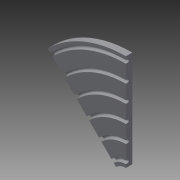
# Autodesk Inventor part: Curved Track Builder
Saved by Autodesk Inventor 2015 SP1 (Build 190203100, 203)
## iProperties
Created: 2015-05-26
Part Number: Curved Track Builder
Material: Generic
Document SubType Name: Modeling
Designer: Andrew
Density: 1 g/cm^3
Appearance: Default
Author: Andrew
Autodesk Inventor part; units mm, degrees
ref_plane "YZ Plane" through (0, 0, 0) normal (1, 0, 0) x (0, 1, 0)
ref_plane "XZ Plane" through (0, 0, 0) normal (0, 1, 0) x (-1, 0, 0)
ref_plane "XY Plane" through (0, 0, 0) normal (0, 0, 1) x (1, 0, 0)
sketch "Sketch1" plane through (0, 0, 0) normal (0, 1, 0) x (-1, 0, 0)
  arc A0 (77.046154, 77.046154) -> (0, 108.959716) centre (0, 0) ccw
  arc A1 (64.375202, 64.375202) -> (0, 91.040284) centre (0, 0) ccw
  line L0 (0, 113.959716) -> (0, 0)
  arc A2 (51.70425, 51.70425) -> (0, 73.120851) centre (0, 0) ccw
  arc A3 (39.033297, 39.033297) -> (0, 55.201418) centre (0, 0) ccw
  arc A4 (26.362345, 26.362345) -> (0, 37.281986) centre (0, 0) ccw
  arc A5 (70.710678, 70.710678) -> (0, 100) centre (0, 0) ccw construction
  arc A6 (13.691392, 13.691392) -> (0, 19.362553) centre (0, 0) ccw
  line L1 (0, 0) -> (80.581688, 80.581688)
  arc A7 (80.581688, 80.581688) -> (0, 113.959716) centre (0, 0) ccw
  arc A8 (10.155859, 10.155859) -> (0, 14.362553) centre (0, 0) ccw
  dimension "d8" = 45
  dimension "d0" = 17.91943
  dimension "d2" = 8.95972
  dimension "d3" = 200
  dimension "d4" = 17.91943
  dimension "d5" = 17.91943
  dimension "d6" = 17.91943
  dimension "d9" = 17.91943
  dimension "d10" = 5
  dimension "d11" = 5
  constraints: 18 point on circle, 9 centre point, 9 coincident, 21 other
  measures "d0" radial gap between concentric circles of A0 A1
  measures "d2" radial gap between concentric circles of A5 A1
  measures "d3" diameter of A5
  measures "d4" radial gap between concentric circles of A2 A1
  measures "d5" radial gap between concentric circles of A3 A2
  measures "d6" radial gap between concentric circles of A3 A4
  measures "d9" radial gap between concentric circles of A6 A4
  measures "d10" radial gap between concentric circles of A8 A6
  measures "d11" radial gap between concentric circles of A7 A0
extrude "Extrusion1" add sketch "Sketch1" along normal blind 5 contours L1 A1 L0 A0 | A0 L0 A7 L1 | L1 A2 L0 A1 | L1 A3 L0 A2 | L1 A4 L0 A3 | L1 A6 L0 A4 | L1 A8 L0 A6
sketch "Sketch2" plane through (-80.581688, 0, 80.581688) normal (-0.7071068, 0, -0.7071068) x (-0.7071068, 0, 0.7071068)
  line L0 (-5, 0) -> (-36.913562, 0)
  line L1 (-22.919433, 0) -> (-49.584514, 0)
  line L2 (-40.838865, 0) -> (-62.255467, 0)
  line L3 (-58.758298, 0) -> (-74.926419, 0)
  line L4 (-76.677731, 0) -> (-87.597372, 0)
  line L5 (-94.597164, 0) -> (-100.268324, 0)
  circle A0 centre (-5, 0) radius 1.65
  circle A1 centre (-22.919433, 0) radius 1.65
  circle A2 centre (-40.838865, 0) radius 1.65
  circle A3 centre (-58.758298, 0) radius 1.65
  circle A4 centre (-76.677731, 0) radius 1.65
  circle A5 centre (-94.597164, 0) radius 1.65
  point P0 (-113.959716, 0)
  dimension "d14" = 3.3
  constraints: 6 centre point, 6 coincident, 5 equal radius
  measures "d14" diameter of A0
sweep "Sweep1" cut profiles "Sketch2" path "Sketch1" path curves A0 contours A0
sweep "Sweep2" cut profiles "Sketch2" path "Sketch1" path curves A1 contours A1 L0 | L0 A1
sweep "Sweep3" cut profiles "Sketch2" path "Sketch1" path curves A2 contours A2 L1 | L1 A2
sweep "Sweep4" cut profiles "Sketch2" path "Sketch1" path curves A3 contours A3 L2 | L2 A3
sweep "Sweep5" cut profiles "Sketch2" path "Sketch1" path curves A4 contours A4
sweep "Sweep6" cut profiles "Sketch2" path "Sketch1" path curves A6 contours A5
sketch "Sketch3" plane through (0, 0, 0) normal (0, -1, 0) x (1, 0, 0)
  arc A0 (0, 110.609716) -> (-78.21288, 78.21288) centre (0, 0) ccw
  line L0 (0, 113.959716) -> (0, 110.609716)
  arc A1 (0, 113.959716) -> (-80.581688, 80.581688) centre (0, 0) ccw
  line L1 (-78.21288, 78.21288) -> (-80.581688, 80.581688)
  arc A2 (0, 92.690284) -> (-65.541928, 65.541928) centre (0, 0) ccw
  line L2 (0, 107.309716) -> (0, 92.690284)
  arc A3 (0, 107.309716) -> (-75.879428, 75.879428) centre (0, 0) ccw
  line L3 (-65.541928, 65.541928) -> (-75.879428, 75.879428)
  arc A4 (0, 74.770851) -> (-52.870976, 52.870976) centre (0, 0) ccw
  line L4 (0, 89.390284) -> (0, 74.770851)
  arc A5 (0, 89.390284) -> (-63.208476, 63.208476) centre (0, 0) ccw
  line L5 (-52.870976, 52.870976) -> (-63.208476, 63.208476)
  arc A6 (0, 56.851418) -> (-40.200023, 40.200023) centre (0, 0) ccw
  line L6 (0, 71.470851) -> (0, 56.851418)
  arc A7 (0, 71.470851) -> (-50.537523, 50.537523) centre (0, 0) ccw
  line L7 (-40.200023, 40.200023) -> (-50.537523, 50.537523)
  arc A8 (0, 38.931986) -> (-27.529071, 27.529071) centre (0, 0) ccw
  line L8 (0, 53.551418) -> (0, 38.931986)
  arc A9 (0, 53.551418) -> (-37.866571, 37.866571) centre (0, 0) ccw
  line L9 (-27.529071, 27.529071) -> (-37.866571, 37.866571)
  arc A10 (0, 21.012553) -> (-14.858119, 14.858119) centre (0, 0) ccw
  line L10 (0, 35.631986) -> (0, 21.012553)
  arc A11 (0, 35.631986) -> (-25.195619, 25.195619) centre (0, 0) ccw
  line L11 (-14.858119, 14.858119) -> (-25.195619, 25.195619)
  arc A12 (0, 17.712553) -> (-12.524666, 12.524666) centre (0, 0) ccw
  line L12 (-10.155859, 10.155859) -> (-12.524666, 12.524666)
  arc A13 (0, 14.362553) -> (-10.155859, 10.155859) centre (0, 0) ccw
  line L13 (0, 17.712553) -> (0, 14.362553)
extrude "Extrusion2" add sketch "Sketch3" along normal blind 1.65
equation "\"d0\" = d25"
equation "\"d2\" = 0.5 * d25"
equation "\"d4\" = d25"
equation "\"d5\" = d4"
equation "\"d6\" = d5"
equation "\"d9\" = d6"
equation "\"d14\" = trackDiameter"
equation "\"d28\" = 0.5 * trackDiameter"
equation "\"d25\" = 17.919433"
equation "\"trackDiameter\" = 3.3"
body "Solid1"
